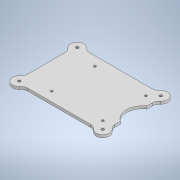
# Autodesk Inventor part: plate_mounting
Saved by Autodesk Inventor 2020 (Build 240168000, 168)
## iProperties
Created: 2020-06-03
Part Number: plate_mounting
Material: Generic
Document SubType Name: Modeling
Designer: suhren
Density: 1 g/cm^3
Appearance: Default
Author: suhren
Autodesk Inventor part; units mm, degrees
ref_plane "YZ Plane" through (0, 0, 0) normal (1, 0, 0) x (0, 1, 0)
ref_plane "XZ Plane" through (0, 0, 0) normal (0, 1, 0) x (-1, 0, 0)
ref_plane "XY Plane" through (0, 0, 0) normal (0, 0, 1) x (1, 0, 0)
sketch "Sketch1" plane through (0, 0, 0) normal (0, 1, 0) x (-1, 0, 0)
  line L0 (-39, -24.5) -> (19, -24.5) construction
  line L1 (19, -24.5) -> (19, 24.5) construction
  line L2 (19, 24.5) -> (-39, 24.5) construction
  line L3 (-39, 24.5) -> (-39, -24.5) construction
  line L4 (42.5, -28) -> (-42.5, -28) construction
  line L5 (-42.5, -28) -> (-42.5, 28) construction
  line L6 (-42.5, 28) -> (42.5, 28) construction
  line L7 (42.5, 28) -> (42.5, -28) construction
  line L8 (50, 0) -> (-50, 0) construction
  line L9 (47.5, -33) -> (-47.5, -33) construction
  line L10 (-47.5, -33) -> (-47.5, 33) construction
  line L11 (-47.5, 33) -> (47.5, 33) construction
  line L12 (47.5, 33) -> (47.5, -33) construction
  circle A0 centre (47.5, -33) radius 7.5
  circle A1 centre (47.5, 33) radius 7.5
  circle A2 centre (-47.5, 33) radius 7.5
  circle A3 centre (-47.5, -33) radius 7.5
  line L13 (49.5, -25.7716) -> (49.5, 25.7716)
  line L14 (40.2716, 35) -> (-40.2716, 35)
  line L15 (-49.5, 25.7716) -> (-49.5, -25.7716)
  line L16 (-40.2716, -35) -> (40.2716, -35)
  arc A4 (-49.5, -15) -> (-49.5, 15) centre (-59.5625, 0) ccw
  point P0 (0, 0)
  point P1 (-39, 0)
  point P2 (0, 0)
  point P3 (0, -28)
  point P4 (0, 0)
  point P5 (0, -33)
  point P6 (-47.5, 0)
  point P7 (-41.5, 0)
  dimension "d0" = 58
  dimension "d1" = 49
  dimension "d2" = 3.5
  dimension "d3" = 3.5
  dimension "d25" = 5
  dimension "d26" = 5
  dimension "d27" = 15
  dimension "d28" = 85
  dimension "d29" = 2
  dimension "d30" = 2
  dimension "d32" = 30
  dimension "d33" = 8
  constraints: 34 end point, 11 point on circle, 7 parallel, 6 coincident, 5 centre point, 5 midpoint, 4 horizontal alignment, 4 perpendicular, 4 vertical alignment, 3 equal radius, 3 horizontal, 2 point on line, 2 vertical, 1 symmetric about line, 1 other
  measures "d0" distance of L0.start L0.end
  measures "d1" distance of L2.end L0.start
  measures "d2" distance between parallel lines of L4 L0
  measures "d3" distance between parallel lines of L5 L3
  measures "d25" horizontal distance of L9.start L4.start
  measures "d26" horizontal distance of L4.start L9.start
  measures "d27" diameter of A0
  measures "d28" distance of L5.end L6.end
  measures "d29" distance between parallel lines of L12 L13
  measures "d30" distance between parallel lines of L9 L16
  measures "d32" distance of A4.end A4.start
  measures "d33" distance from line of L15 point (-41.5, 0)
extrude "Extrusion1" add sketch "Sketch1" along normal blind 3 contours A0 | A0 L16 A3 L15 A4 A2 L14 A1 L13 | A1 | A3 | A2
fillet "Fillet2" radius 8 8 edges at (-49.5, 1.5, -25.7716) (-49.5, 1.5, 25.7716) (-40.2716, 1.5, 35) (40.2716, 1.5, 35) (49.5, 1.5, 25.7716) (49.5, 1.5, -25.7716) (40.2716, 1.5, -35) (-40.2716, 1.5, -35)
hole "Hole1" at (-47.5, 0, 33) at (-47.5, 0, -33) at (47.5, 0, -33) at (47.5, 0, 33) direction (0, 1, 0) diameter 3 end through all
hole "Hole2" at (-19, 0, 24.5) at (-19, 0, -24.5) at (39, 0, -24.5) at (39, 0, 24.5) direction (0, 1, 0) diameter 2.5 end through all
sketch "Sketch3" plane through (0, 3, 0) normal (0, 1, 0) x (1, 0, 0)
  circle A0 centre (39, 24.5) radius 1.25 projected
  circle A1 centre (-19, -24.5) radius 1.25 projected
  circle A2 centre (-19, 24.5) radius 1.25 projected
  circle A3 centre (39, -24.5) radius 1.25 projected
  circle A4 centre (47.5, 33) radius 1.5 projected
  circle A5 centre (-47.5, -33) radius 1.5 projected
  circle A6 centre (-47.5, 33) radius 1.5 projected
  circle A7 centre (47.5, -33) radius 1.5 projected
  line L0 (49.5, 15) -> (49.5, 21.1573) projected
  arc A8 (52.3387, 27.2697) -> (49.5, 21.1573) centre (57.5, 21.1573) ccw projected
  arc A9 (52.3387, 27.2697) -> (41.7697, 37.8387) centre (47.5, 33) ccw projected
  arc A10 (35.6573, 35) -> (41.7697, 37.8387) centre (35.6573, 43) ccw projected
  line L1 (35.6573, 35) -> (-35.6573, 35) projected
  arc A11 (-41.7697, 37.8387) -> (-35.6573, 35) centre (-35.6573, 43) ccw projected
  arc A12 (-41.7697, 37.8387) -> (-52.3387, 27.2697) centre (-47.5, 33) ccw projected
  arc A13 (-49.5, 21.1573) -> (-52.3387, 27.2697) centre (-57.5, 21.1573) ccw projected
  line L2 (-49.5, 21.1573) -> (-49.5, -21.1573) projected
  arc A14 (-52.3387, -27.2697) -> (-49.5, -21.1573) centre (-57.5, -21.1573) ccw projected
  arc A15 (-52.3387, -27.2697) -> (-41.7697, -37.8387) centre (-47.5, -33) ccw projected
  arc A16 (-35.6573, -35) -> (-41.7697, -37.8387) centre (-35.6573, -43) ccw projected
  line L3 (-35.6573, -35) -> (35.6573, -35) projected
  arc A17 (41.7697, -37.8387) -> (35.6573, -35) centre (35.6573, -43) ccw projected
  arc A18 (41.7697, -37.8387) -> (52.3387, -27.2697) centre (47.5, -33) ccw projected
  arc A19 (49.5, -21.1573) -> (52.3387, -27.2697) centre (57.5, -21.1573) ccw projected
  line L4 (49.5, -21.1573) -> (49.5, -15) projected
  arc A20 (49.5, 15) -> (49.5, -15) centre (59.5625, 0) ccw projected
  point P0 (0, 0)
equation "\"d3\" = d2"
equation "\"d26\" = d25"
equation "\"d30\" = d29"
body "Solid1"
